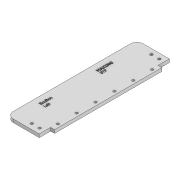
# Autodesk Inventor part: Comb2
Saved by Autodesk Inventor 2020 (Build 240168000, 168)
## iProperties
Created: 2022-04-26
Part Number: Comb2
Material: Generic
Document SubType Name: Modeling
Designer: ferrerx
Density: 1 g/cm^3
Appearance: Default
Author: ferrerx
Autodesk Inventor part; units mm, degrees
ref_plane "YZ Plane" through (0, 0, 0) normal (1, 0, 0) x (0, 1, 0)
ref_plane "XZ Plane" through (0, 0, 0) normal (0, 1, 0) x (-1, 0, 0)
ref_plane "XY Plane" through (0, 0, 0) normal (0, 0, 1) x (1, 0, 0)
sketch "Sketch1" plane through (0, 0, 0) normal (0, 1, 0) x (-1, 0, 0)
  line L0 (25, 100) -> (-25, 100)
  line L1 (-25, 100) -> (-25, -100)
  line L2 (-25, -100) -> (25, -100)
  line L3 (25, -100) -> (25, 100)
  line L4 (25, 100) -> (-25, -100) construction
  line L5 (-25, 100) -> (25, -100) construction
  point P0 (0, 0)
  dimension "d0" = 200
  dimension "d1" = 50
  constraints: 12 end point, 2 midpoint, 2 parallel, 1 horizontal, 1 perpendicular
  measures "d0" distance of L2.end L0.start
  measures "d1" distance of L1.end L2.end
extrude "Extrusion1" add sketch "Sketch1" along normal blind 5
sketch "Sketch2" plane through (0, 5, 0) normal (0, 1, 0) x (1, 0, 0)
  line L0 (0, 0) -> (25, 0) construction
  line L1 (25, -100) -> (25, 100) projected
  line L2 (25, -92) -> (-15.0756, -92) construction
  circle A0 centre (17.5, -92) radius 2
  circle A1 centre (5.5, -92) radius 2
  line L3 (-25, -100) -> (25, -100) projected
  circle A2 centre (17.5, 92) radius 2
  circle A3 centre (5.5, 92) radius 2
  dimension "d4" = 4
  dimension "d5" = 4
  dimension "d6" = 12
  dimension "d7" = 8
  dimension "d10" = 7.5
  constraints: 4 centre point, 4 end point, 3 point on line, 2 symmetric about line, 1 horizontal, 1 midpoint, 2 other
  measures "d4" diameter of A1
  measures "d5" diameter of A0
  measures "d6" distance of A1.centre A0.centre
  measures "d7" distance between parallel lines of L3 L2
  measures "d10" distance from line of L1 A0.centre
extrude "Extrusion2" cut sketch "Sketch2" against normal blind 5
sketch "Sketch3" plane through (0, 5, 0) normal (0, 1, 0) x (1, 0, 0)
  line L0 (19, -82.5) -> (31, -82.5)
  line L1 (31, -82.5) -> (31, 82.5)
  line L2 (31, 82.5) -> (19, 82.5)
  line L3 (19, 82.5) -> (19, -82.5)
  line L4 (25, -100) -> (25, 100) projected
  line L5 (19, -82.5) -> (31, 82.5) construction
  line L6 (31, -82.5) -> (19, 82.5) construction
  point P0 (0, 0)
  point P1 (25, 0)
  dimension "d11" = 165
  dimension "d12" = 12
  constraints: 12 end point, 3 midpoint, 2 parallel, 1 horizontal, 1 perpendicular
  measures "d11" distance of L0.end L1.end
  measures "d12" distance of L1.end L2.end
extrude "Extrusion3" add sketch "Sketch3" against normal blind 5
sketch "Sketch4" plane through (0, 5, 0) normal (0, 1, 0) x (1, 0, 0)
  line L0 (25, -100) -> (25, -82.5) projected
  line L1 (31, 82.5) -> (25, 82.5) projected
  circle A0 centre (26, -72.5) radius 2
  line L2 (25, -82.5) -> (31, -82.5) projected
  line L3 (31, -82.5) -> (31, 82.5) projected
  point P0 (0, 0)
  dimension "d15" = 4
  dimension "d16" = 10
  dimension "d17" = 5
  constraints: 1 centre point
  measures "d15" diameter of A0
  measures "d16" distance from line of L2 A0.centre
  measures "d17" distance from line of L3 A0.centre
extrude "Extrusion4" cut sketch "Sketch4" against normal blind 5
pattern_linear "Rectangular Pattern1" count 6 spacing 29 along (0, 0, -1) of "Extrusion4"
fillet "Fillet1" radius 10 2 edges at (-25, 2.5, -100) (-25, 2.5, 100)
sketch "Sketch5" plane through (0, 5, 0) normal (0, 1, 0) x (1, 0, 0)
  line L0 (14.5574, 78.2537) -> (14.5574, 41.6)
  line L1 (14.5574, 41.6) -> (-22.0963, 41.6)
  line L2 (-22.0963, 41.6) -> (-22.0963, 78.2537)
  line L3 (-22.0963, 60) -> (14.5574, 60)
  line L4 (-22.0387, 23.3375) -> (14.5574, 23.3375)
  line L5 (14.5574, 23.3375) -> (14.5574, 60)
  line L6 (14.5574, 60) -> (-22.0387, 60)
  line L7 (-22.0387, 60) -> (-22.0387, 23.3375)
  line L8 (25, 100) -> (-15, 100) projected
  line L9 (-22.0387, 60) -> (31, 60) construction
  line L10 (31, -82.5) -> (31, 82.5) projected
  line L11 (-12.3449, 32.3329) -> (-12.3449, 31.3043)
  line L12 (-12.3449, 31.3043) -> (-15.0767, 31.3043)
  line L13 (-15.0767, 31.3043) -> (-13.3134, 30.5562)
  line L14 (-13.3134, 30.5562) -> (-13.3134, 29.8482)
  line L15 (-13.3134, 29.8482) -> (-15.0767, 29.1001)
  line L16 (-15.0767, 29.1001) -> (-12.3449, 29.1001)
  line L17 (-12.3449, 29.1001) -> (-12.3449, 28.1249)
  line L18 (-12.3449, 28.1249) -> (-16.466, 28.1249)
  line L19 (-16.466, 28.1249) -> (-16.466, 29.3172)
  line L20 (-16.466, 29.3172) -> (-14.4321, 30.2322)
  line L21 (-14.4321, 30.2322) -> (-16.466, 31.1406)
  line L22 (-16.466, 31.1406) -> (-16.466, 32.3329)
  line L23 (-16.466, 32.3329) -> (-12.3449, 32.3329)
  line L24 (-12.3449, 32.7437) -> (-16.466, 34.1363)
  line L25 (-16.466, 34.1363) -> (-16.466, 35.2651)
  line L26 (-16.466, 35.2651) -> (-12.3449, 36.6578)
  line L27 (-12.3449, 36.6578) -> (-12.3449, 35.5924)
  line L28 (-12.3449, 35.5924) -> (-13.1865, 35.3353)
  line L29 (-13.1865, 35.3353) -> (-13.1865, 34.0395)
  line L30 (-13.1865, 34.0395) -> (-12.3449, 33.779)
  line L31 (-12.3449, 33.779) -> (-12.3449, 32.7437)
  line L32 (-13.9345, 35.1082) -> (-15.2971, 34.6874)
  line L33 (-15.2971, 34.6874) -> (-13.9345, 34.2632)
  line L34 (-13.9345, 34.2632) -> (-13.9345, 35.1082)
  line L35 (-12.3449, 40.6787) -> (-12.3449, 39.4263)
  line L36 (-12.3449, 39.4263) -> (-14.018, 38.3076)
  line L37 (-14.018, 38.3076) -> (-13.7375, 38.1038)
  line L38 (-13.7375, 38.1038) -> (-12.3449, 38.1038)
  line L39 (-12.3449, 38.1038) -> (-12.3449, 37.0685)
  line L40 (-12.3449, 37.0685) -> (-16.466, 37.0685)
  line L41 (-16.466, 37.0685) -> (-16.466, 38.1038)
  line L42 (-16.466, 38.1038) -> (-14.6258, 38.1038)
  line L43 (-14.6258, 38.1038) -> (-16.466, 39.4263)
  line L44 (-16.466, 39.4263) -> (-16.466, 40.6186)
  line L45 (-16.466, 40.6186) -> (-14.5524, 39.1492)
  line L46 (-14.5524, 39.1492) -> (-12.3449, 40.6787)
  line L47 (-12.3449, 43.0666) -> (-12.3449, 40.849)
  line L48 (-12.3449, 40.849) -> (-13.0629, 40.849)
  line L49 (-13.0629, 40.849) -> (-13.0629, 41.4402)
  line L50 (-13.0629, 41.4402) -> (-15.748, 41.4402)
  line L51 (-15.748, 41.4402) -> (-15.748, 40.849)
  line L52 (-15.748, 40.849) -> (-16.466, 40.849)
  line L53 (-16.466, 40.849) -> (-16.466, 43.0666)
  line L54 (-16.466, 43.0666) -> (-15.748, 43.0666)
  line L55 (-15.748, 43.0666) -> (-15.748, 42.4755)
  line L56 (-15.748, 42.4755) -> (-13.0629, 42.4755)
  line L57 (-13.0629, 42.4755) -> (-13.0629, 43.0666)
  line L58 (-13.0629, 43.0666) -> (-12.3449, 43.0666)
  line L59 (-12.3449, 47.2846) -> (-12.3449, 46.2894)
  line L60 (-12.3449, 46.2894) -> (-15.217, 44.6997)
  line L61 (-15.217, 44.6997) -> (-12.3449, 44.6997)
  line L62 (-12.3449, 44.6997) -> (-12.3449, 43.7546)
  line L63 (-12.3449, 43.7546) -> (-16.466, 43.7546)
  line L64 (-16.466, 43.7546) -> (-16.466, 45.0236)
  line L65 (-16.466, 45.0236) -> (-14.1049, 46.3395)
  line L66 (-14.1049, 46.3395) -> (-16.466, 46.3395)
  line L67 (-16.466, 46.3395) -> (-16.466, 47.2846)
  line L68 (-16.466, 47.2846) -> (-12.3449, 47.2846)
  spline S0 degree 2 poles (-12.5786, 51.5627) (-12.4684, 51.2922) (-12.258, 50.4272) (-12.258, 50.0064) knots 0 0 0 1 2 2 2
  spline S1 degree 2 poles (-12.258, 50.0064) (-12.258, 49.0346) (-13.3802, 47.8824) (-14.4088, 47.8824) knots 0 0 0 1 2 2 2
  spline S2 degree 2 poles (-14.4088, 47.8824) (-15.3773, 47.8824) (-16.5462, 49.0346) (-16.5462, 50.0365) knots 0 0 0 1 2 2 2
  spline S3 degree 2 poles (-16.5462, 50.0365) (-16.5462, 50.5541) (-16.3491, 51.202) (-16.1821, 51.546) knots 0 0 0 1 2 2 2
  line L69 (-16.1821, 51.546) -> (-15.2136, 51.546)
  line L70 (-15.2136, 51.546) -> (-15.2136, 51.4525)
  spline S4 degree 2 poles (-15.2136, 51.4525) (-15.2704, 51.379) (-15.4875, 51.0985) (-15.561, 50.9649) knots 0 0 0 1 2 2 2
  spline S5 degree 2 poles (-15.561, 50.9649) (-15.6511, 50.8113) (-15.778, 50.4038) (-15.778, 50.1767) knots 0 0 0 1 2 2 2
  spline S6 degree 2 poles (-15.778, 50.1767) (-15.778, 49.9129) (-15.6111, 49.4754) (-15.4407, 49.3051) knots 0 0 0 1 2 2 2
  spline S7 degree 2 poles (-15.4407, 49.3051) (-15.2737, 49.1414) (-14.7628, 48.9511) (-14.4255, 48.9511) knots 0 0 0 1 2 2 2
  spline S8 degree 2 poles (-14.4255, 48.9511) (-13.7041, 48.9511) (-13.0161, 49.6758) (-13.0161, 50.3003) knots 0 0 0 1 2 2 2
  spline S9 degree 2 poles (-13.0161, 50.3003) (-13.0161, 50.3571) (-13.0228, 50.504) (-13.0261, 50.5608) knots 0 0 0 1 2 2 2
  line L71 (-13.0261, 50.5608) -> (-13.8377, 50.5608)
  line L72 (-13.8377, 50.5608) -> (-13.8377, 49.7626)
  line L73 (-13.8377, 49.7626) -> (-14.6092, 49.7626)
  line L74 (-14.6092, 49.7626) -> (-14.6092, 51.5627)
  line L75 (-14.6092, 51.5627) -> (-12.5786, 51.5627)
  spline S10 degree 2 poles (-6.6136, 29.2163) (-6.6136, 28.7823) (-6.7949, 28.1735) (-6.9245, 27.9047) knots 0 0 0 1 2 2 2
  line L76 (-6.9245, 27.9047) -> (-7.5916, 27.9047)
  line L77 (-7.5916, 27.9047) -> (-7.5916, 27.9436)
  spline S11 degree 2 poles (-7.5916, 27.9436) (-7.3455, 28.2059) (-7.0734, 28.8698) (-7.0734, 29.1774) knots 0 0 0 1 2 2 2
  spline S12 degree 2 poles (-7.0734, 29.1774) (-7.0734, 29.6178) (-7.4394, 30.068) (-7.7406, 30.068) knots 0 0 0 1 2 2 2
  spline S13 degree 2 poles (-7.7406, 30.068) (-7.9802, 30.068) (-8.2782, 29.8316) (-8.3526, 29.5757) knots 0 0 0 1 2 2 2
  spline S14 degree 2 poles (-8.3526, 29.5757) (-8.4045, 29.3912) (-8.4757, 29.0835) (-8.534, 28.8536) knots 0 0 0 1 2 2 2
  spline S15 degree 2 poles (-8.534, 28.8536) (-8.589, 28.6463) (-8.7542, 28.3192) (-8.887, 28.1929) knots 0 0 0 1 2 2 2
  spline S16 degree 2 poles (-8.887, 28.1929) (-9.0198, 28.0699) (-9.376, 27.9338) (-9.6092, 27.9338) knots 0 0 0 1 2 2 2
  spline S17 degree 2 poles (-9.6092, 27.9338) (-10.0949, 27.9338) (-10.7523, 28.6916) (-10.7523, 29.2778) knots 0 0 0 1 2 2 2
  spline S18 degree 2 poles (-10.7523, 29.2778) (-10.7523, 29.6146) (-10.6196, 30.2105) (-10.4933, 30.4663) knots 0 0 0 1 2 2 2
  line L78 (-10.4933, 30.4663) -> (-9.8585, 30.4663)
  line L79 (-9.8585, 30.4663) -> (-9.8585, 30.4275)
  spline S19 degree 2 poles (-9.8585, 30.4275) (-10.0334, 30.2364) (-10.2925, 29.6405) (-10.2925, 29.3134) knots 0 0 0 1 2 2 2
  spline S20 degree 2 poles (-10.2925, 29.3134) (-10.2925, 28.9442) (-9.946, 28.4876) (-9.6642, 28.4876) knots 0 0 0 1 2 2 2
  spline S21 degree 2 poles (-9.6642, 28.4876) (-9.4116, 28.4876) (-9.1104, 28.7564) (-9.0424, 29.009) knots 0 0 0 1 2 2 2
  spline S22 degree 2 poles (-9.0424, 29.009) (-8.9971, 29.1774) (-8.8805, 29.6664) (-8.8319, 29.8283) knots 0 0 0 1 2 2 2
  spline S23 degree 2 poles (-8.8319, 29.8283) (-8.7056, 30.2396) (-8.1972, 30.6218) (-7.8248, 30.6218) knots 0 0 0 1 2 2 2
  spline S24 degree 2 poles (-7.8248, 30.6218) (-7.5884, 30.6218) (-7.135, 30.4307) (-6.9763, 30.2591) knots 0 0 0 1 2 2 2
  spline S25 degree 2 poles (-6.9763, 30.2591) (-6.8014, 30.068) (-6.6136, 29.5822) (-6.6136, 29.2163) knots 0 0 0 1 2 2 2
  line L80 (-6.6848, 32.0953) -> (-10.2083, 32.0953)
  line L81 (-10.2083, 32.0953) -> (-10.2083, 30.7545)
  line L82 (-10.2083, 30.7545) -> (-10.6811, 30.7545)
  line L83 (-10.6811, 30.7545) -> (-10.6811, 33.9671)
  line L84 (-10.6811, 33.9671) -> (-10.2083, 33.9671)
  line L85 (-10.2083, 33.9671) -> (-10.2083, 32.6264)
  line L86 (-10.2083, 32.6264) -> (-6.6848, 32.6264)
  line L87 (-6.6848, 32.6264) -> (-6.6848, 32.0953)
  spline S26 degree 2 poles (-9.4764, 36.8979) (-9.2173, 36.8979) (-8.751, 36.7133) (-8.589, 36.5482) knots 0 0 0 1 2 2 2
  spline S27 degree 2 poles (-8.589, 36.5482) (-8.385, 36.3409) (-8.1745, 35.7806) (-8.1745, 35.3532) knots 0 0 0 1 2 2 2
  line L88 (-8.1745, 35.3532) -> (-8.1745, 34.903)
  line L89 (-8.1745, 34.903) -> (-6.6848, 34.903)
  line L90 (-6.6848, 34.903) -> (-6.6848, 34.3719)
  line L91 (-6.6848, 34.3719) -> (-10.6811, 34.3719)
  line L92 (-10.6811, 34.3719) -> (-10.6811, 35.3758)
  spline S28 degree 2 poles (-10.6811, 35.3758) (-10.6811, 35.7321) (-10.5645, 36.2308) (-10.4317, 36.4219) knots 0 0 0 1 2 2 2
  spline S29 degree 2 poles (-10.4317, 36.4219) (-10.2795, 36.6453) (-9.8099, 36.8979) (-9.4764, 36.8979) knots 0 0 0 1 2 2 2
  spline S30 degree 2 poles (-9.4602, 36.3441) (-9.6675, 36.3441) (-9.9719, 36.2016) (-10.069, 36.0559) knots 0 0 0 1 2 2 2
  spline S31 degree 2 poles (-10.069, 36.0559) (-10.1532, 35.9296) (-10.2212, 35.5928) (-10.2212, 35.3435) knots 0 0 0 1 2 2 2
  line L93 (-10.2212, 35.3435) -> (-10.2212, 34.903)
  line L94 (-10.2212, 34.903) -> (-8.6279, 34.903)
  line L95 (-8.6279, 34.903) -> (-8.6279, 35.2657)
  spline S32 degree 2 poles (-8.6279, 35.2657) (-8.6279, 35.5896) (-8.7315, 35.9879) (-8.8676, 36.1174) knots 0 0 0 1 2 2 2
  spline S33 degree 2 poles (-8.8676, 36.1174) (-8.9874, 36.2373) (-9.2691, 36.3441) (-9.4602, 36.3441) knots 0 0 0 1 2 2 2
  point P0 (0, 0)
  point P1 (-12.258, 27.6974)
  point P2 (-6.6136, 27.6974)
  dimension "d33" = 40
  constraints: 18 end point, 2 horizontal, 2 parallel, 1 perpendicular, 1 point on line, 2 other
  measures "d33" distance between parallel lines of L8 L3
emboss "Emboss1" sketch "Sketch5" operation cut depth 1 direction (0, -1, 0) contours L47 L48 L49 L50 L51 L52 L53 L1 | L1 L53 L54 L55 L56 L57 L58 L47 | L11 L12 L13 L14 L15 L16 L17 L18 L19 L20 L21 L22 L23 | L24 L25 L26 L27 L28 L29 L30 L31 | L35 L36 L37 L38 L39 L40 L41 L42 L43 L44 L45 L46 | L59 L60 L61 L62 L63 L64 L65 L66 L67 L68 | S0 S1 S2 S3 L69 L70 S4 S5 S6 S7 S8 S9 L71 L72 L73 L74 L75 | S10 L76 L77 S11 S12 S13 S14 S15 S16 S17 S18 L78 L79 S19 S20 S21 S22 S23 S24 S25 | L80 L81 L82 L83 L84 L85 L86 L87 | S26 S27 L88 L89 L90 L91 L92 S28 S29
sketch "Sketch6" plane through (0, 5, 0) normal (0, 1, 0) x (1, 0, 0)
  line L0 (-16.466, -60) -> (-16.394, -19.5573) construction
  line L1 (-16.394, -19.5573) -> (0.0633, -19.5866) construction
  line L2 (0.0633, -19.5866) -> (-0.0087, -60.0293) construction
  line L3 (-0.0087, -60.0293) -> (-16.466, -60) construction
  line L4 (-12.3449, 28.1249) -> (-16.466, 28.1249) projected
  line L5 (-16.466, -60) -> (-16.466, 28.1249) construction
  line L6 (31, -82.5) -> (31, 82.5) projected
  line L7 (-15, -100) -> (25, -100) projected
  line L8 (-16.466, -60) -> (31, -60) construction
  spline S0 degree 2 poles (-13.5135, -56.8898) (-13.2155, -56.8904) (-12.7593, -57.1179) (-12.6107, -57.306) knots 0 0 0 1 2 2 2
  spline S1 degree 2 poles (-12.6107, -57.306) (-12.4362, -57.533) (-12.2881, -58.0482) (-12.2889, -58.4562) knots 0 0 0 1 2 2 2
  line L9 (-12.2889, -58.4562) -> (-12.2909, -59.6026)
  line L10 (-12.2909, -59.6026) -> (-16.2872, -59.5955)
  line L11 (-16.2872, -59.5955) -> (-16.2853, -58.5365)
  spline S2 degree 2 poles (-16.2853, -58.5365) (-16.2845, -58.1091) (-16.2287, -57.6817) (-16.1215, -57.4876) knots 0 0 0 1 2 2 2
  spline S3 degree 2 poles (-16.1215, -57.4876) (-16.0078, -57.2708) (-15.635, -57.0739) (-15.3824, -57.0744) knots 0 0 0 1 2 2 2
  spline S4 degree 2 poles (-15.3824, -57.0744) (-15.1006, -57.0749) (-14.6543, -57.3736) (-14.5284, -57.6361) knots 0 0 0 1 2 2 2
  line L12 (-14.5284, -57.6361) -> (-14.509, -57.6362)
  spline S5 degree 2 poles (-14.509, -57.6362) (-14.4112, -57.2801) (-13.8956, -56.8892) (-13.5135, -56.8898) knots 0 0 0 1 2 2 2
  spline S6 degree 2 poles (-13.4918, -57.4437) (-13.7185, -57.4433) (-14.0102, -57.5723) (-14.1141, -57.7664) knots 0 0 0 1 2 2 2
  spline S7 degree 2 poles (-14.1141, -57.7664) (-14.1791, -57.8926) (-14.2185, -58.1905) (-14.219, -58.4657) knots 0 0 0 1 2 2 2
  line L13 (-14.219, -58.4657) -> (-14.2201, -59.0681)
  line L14 (-14.2201, -59.0681) -> (-12.7433, -59.0707)
  line L15 (-12.7433, -59.0707) -> (-12.7426, -58.64)
  spline S8 degree 2 poles (-12.7426, -58.64) (-12.742, -58.2902) (-12.806, -57.8886) (-12.9094, -57.7329) knots 0 0 0 1 2 2 2
  spline S9 degree 2 poles (-12.9094, -57.7329) (-13.016, -57.5838) (-13.2813, -57.444) (-13.4918, -57.4437) knots 0 0 0 1 2 2 2
  spline S10 degree 2 poles (-15.3089, -57.6283) (-15.4514, -57.628) (-15.6653, -57.7248) (-15.727, -57.8315) knots 0 0 0 1 2 2 2
  spline S11 degree 2 poles (-15.727, -57.8315) (-15.7985, -57.961) (-15.8314, -58.275) (-15.8319, -58.5568) knots 0 0 0 1 2 2 2
  line L16 (-15.8319, -58.5568) -> (-15.8328, -59.0652)
  line L17 (-15.8328, -59.0652) -> (-14.6638, -59.0673)
  line L18 (-14.6638, -59.0673) -> (-14.6627, -58.4649)
  spline S12 degree 2 poles (-14.6627, -58.4649) (-14.6622, -58.2156) (-14.7136, -57.9791) (-14.7944, -57.8526) knots 0 0 0 1 2 2 2
  spline S13 degree 2 poles (-14.7944, -57.8526) (-14.8719, -57.7294) (-15.1211, -57.6286) (-15.3089, -57.6283) knots 0 0 0 1 2 2 2
  spline S14 degree 2 poles (-13.7802, -53.9359) (-13.0224, -53.9372) (-12.1979, -54.6674) (-12.199, -55.2762) knots 0 0 0 1 2 2 2
  spline S15 degree 2 poles (-12.199, -55.2762) (-12.2001, -55.9012) (-13.0531, -56.6154) (-13.785, -56.6141) knots 0 0 0 1 2 2 2
  spline S16 degree 2 poles (-13.785, -56.6141) (-14.5363, -56.6128) (-15.3673, -55.8729) (-15.3662, -55.2706) knots 0 0 0 1 2 2 2
  spline S17 degree 2 poles (-15.3662, -55.2706) (-15.3651, -54.6617) (-14.5348, -53.9345) (-13.7802, -53.9359) knots 0 0 0 1 2 2 2
  spline S18 degree 2 poles (-13.7812, -54.4573) (-14.3641, -54.4562) (-14.9316, -54.8795) (-14.9323, -55.2713) knots 0 0 0 1 2 2 2
  spline S19 degree 2 poles (-14.9323, -55.2713) (-14.933, -55.6632) (-14.367, -56.0917) (-13.7841, -56.0927) knots 0 0 0 1 2 2 2
  spline S20 degree 2 poles (-13.7841, -56.0927) (-13.2173, -56.0937) (-12.6337, -55.6673) (-12.633, -55.2754) knots 0 0 0 1 2 2 2
  spline S21 degree 2 poles (-12.633, -55.2754) (-12.6323, -54.8868) (-13.2047, -54.4583) (-13.7812, -54.4573) knots 0 0 0 1 2 2 2
  line L19 (-12.2758, -51.0887) -> (-12.2767, -51.5939)
  line L20 (-12.2767, -51.5939) -> (-12.607, -51.5933)
  spline S22 degree 2 poles (-12.607, -51.5933) (-12.4034, -51.8269) (-12.1936, -52.245) (-12.1941, -52.5041) knots 0 0 0 1 2 2 2
  spline S23 degree 2 poles (-12.1941, -52.5041) (-12.1944, -52.6984) (-12.3246, -53.0447) (-12.4641, -53.1707) knots 0 0 0 1 2 2 2
  spline S24 degree 2 poles (-12.4641, -53.1707) (-12.6035, -53.3) (-13.028, -53.4417) (-13.3324, -53.4412) knots 0 0 0 1 2 2 2
  line L21 (-13.3324, -53.4412) -> (-15.2788, -53.4377)
  line L22 (-15.2788, -53.4377) -> (-15.2779, -52.9325)
  line L23 (-15.2779, -52.9325) -> (-13.568, -52.9356)
  spline S25 degree 2 poles (-13.568, -52.9356) (-13.3283, -52.936) (-13.0141, -52.9009) (-12.8974, -52.8396) knots 0 0 0 1 2 2 2
  spline S26 degree 2 poles (-12.8974, -52.8396) (-12.7807, -52.7783) (-12.6735, -52.568) (-12.6731, -52.3704) knots 0 0 0 1 2 2 2
  spline S27 degree 2 poles (-12.6731, -52.3704) (-12.6728, -52.1858) (-12.8826, -51.7677) (-13.0345, -51.5926) knots 0 0 0 1 2 2 2
  line L24 (-13.0345, -51.5926) -> (-15.2755, -51.5886)
  line L25 (-15.2755, -51.5886) -> (-15.2746, -51.0834)
  line L26 (-15.2746, -51.0834) -> (-12.2758, -51.0887)
  line L27 (-12.2735, -49.8419) -> (-12.2744, -50.3471)
  line L28 (-12.2744, -50.3471) -> (-16.4488, -50.3397)
  line L29 (-16.4488, -50.3397) -> (-16.4479, -49.8345)
  line L30 (-16.4479, -49.8345) -> (-12.2735, -49.8419)
  spline S28 degree 2 poles (-12.2123, -48.1936) (-12.213, -48.6049) (-12.6834, -49.0672) (-13.1919, -49.0663) knots 0 0 0 1 2 2 2
  line L31 (-13.1919, -49.0663) -> (-14.8532, -49.0633)
  line L32 (-14.8532, -49.0633) -> (-14.8538, -49.4034)
  line L33 (-14.8538, -49.4034) -> (-15.2716, -49.4026)
  line L34 (-15.2716, -49.4026) -> (-15.271, -49.0626)
  line L35 (-15.271, -49.0626) -> (-16.1324, -49.061)
  line L36 (-16.1324, -49.061) -> (-16.1315, -48.5558)
  line L37 (-16.1315, -48.5558) -> (-15.2701, -48.5574)
  line L38 (-15.2701, -48.5574) -> (-15.2684, -47.6279)
  line L39 (-15.2684, -47.6279) -> (-14.8507, -47.6287)
  line L40 (-14.8507, -47.6287) -> (-14.8523, -48.5581)
  line L41 (-14.8523, -48.5581) -> (-13.4242, -48.5607)
  spline S29 degree 2 poles (-13.4242, -48.5607) (-13.1975, -48.5611) (-12.9481, -48.5453) (-12.8411, -48.4904) knots 0 0 0 1 2 2 2
  spline S30 degree 2 poles (-12.8411, -48.4904) (-12.7471, -48.4453) (-12.6528, -48.2414) (-12.6525, -48.0665) knots 0 0 0 1 2 2 2
  spline S31 degree 2 poles (-12.6525, -48.0665) (-12.6523, -47.9435) (-12.7264, -47.7134) (-12.749, -47.6616) knots 0 0 0 1 2 2 2
  line L42 (-12.749, -47.6616) -> (-12.7489, -47.6324)
  line L43 (-12.7489, -47.6324) -> (-12.2955, -47.6332)
  spline S32 degree 2 poles (-12.2955, -47.6332) (-12.2569, -47.7758) (-12.2121, -48.0673) (-12.2123, -48.1936) knots 0 0 0 1 2 2 2
  spline S33 degree 2 poles (-13.764, -44.7937) (-13.0062, -44.7951) (-12.1817, -45.5252) (-12.1827, -46.134) knots 0 0 0 1 2 2 2
  spline S34 degree 2 poles (-12.1827, -46.134) (-12.1839, -46.759) (-13.0368, -47.4732) (-13.7687, -47.4719) knots 0 0 0 1 2 2 2
  spline S35 degree 2 poles (-13.7687, -47.4719) (-14.5201, -47.4706) (-15.351, -46.7307) (-15.35, -46.1284) knots 0 0 0 1 2 2 2
  spline S36 degree 2 poles (-15.35, -46.1284) (-15.3489, -45.5195) (-14.5185, -44.7924) (-13.764, -44.7937) knots 0 0 0 1 2 2 2
  spline S37 degree 2 poles (-13.7649, -45.3151) (-14.3478, -45.3141) (-14.9153, -45.7373) (-14.916, -46.1291) knots 0 0 0 1 2 2 2
  spline S38 degree 2 poles (-14.916, -46.1291) (-14.9167, -46.521) (-14.3507, -46.9495) (-13.7678, -46.9505) knots 0 0 0 1 2 2 2
  spline S39 degree 2 poles (-13.7678, -46.9505) (-13.2011, -46.9515) (-12.6174, -46.5251) (-12.6167, -46.1332) knots 0 0 0 1 2 2 2
  spline S40 degree 2 poles (-12.6167, -46.1332) (-12.616, -45.7446) (-13.1885, -45.3161) (-13.7649, -45.3151) knots 0 0 0 1 2 2 2
  line L44 (-12.2595, -41.9239) -> (-12.2603, -42.4291)
  line L45 (-12.2603, -42.4291) -> (-13.9703, -42.426)
  spline S41 degree 2 poles (-13.9703, -42.426) (-14.1775, -42.4257) (-14.5338, -42.4639) (-14.6408, -42.522) knots 0 0 0 1 2 2 2
  spline S42 degree 2 poles (-14.6408, -42.522) (-14.7542, -42.5833) (-14.8647, -42.8033) (-14.8651, -42.9912) knots 0 0 0 1 2 2 2
  spline S43 degree 2 poles (-14.8651, -42.9912) (-14.8654, -43.179) (-14.6653, -43.5777) (-14.5038, -43.769) knots 0 0 0 1 2 2 2
  line L46 (-14.5038, -43.769) -> (-12.2627, -43.773)
  line L47 (-12.2627, -43.773) -> (-12.2636, -44.2782)
  line L48 (-12.2636, -44.2782) -> (-15.2625, -44.2729)
  line L49 (-15.2625, -44.2729) -> (-15.2616, -43.7677)
  line L50 (-15.2616, -43.7677) -> (-14.928, -43.7683)
  spline S44 degree 2 poles (-14.928, -43.7683) (-15.1316, -43.5412) (-15.3446, -43.1037) (-15.3441, -42.8575) knots 0 0 0 1 2 2 2
  spline S45 degree 2 poles (-15.3441, -42.8575) (-15.3434, -42.4171) (-14.7595, -41.9194) (-14.2058, -41.9204) knots 0 0 0 1 2 2 2
  line L51 (-14.2058, -41.9204) -> (-12.2595, -41.9239)
  line L52 (-5.7071, -57.2988) -> (-5.7112, -59.6143)
  line L53 (-5.7112, -59.6143) -> (-9.7074, -59.6072)
  line L54 (-9.7074, -59.6072) -> (-9.7065, -59.0761)
  line L55 (-9.7065, -59.0761) -> (-6.183, -59.0824)
  line L56 (-6.183, -59.0824) -> (-6.1799, -57.298)
  line L57 (-6.1799, -57.298) -> (-5.7071, -57.2988)
  spline S46 degree 2 poles (-6.0208, -55.2483) (-5.9755, -55.3099) (-5.814, -55.5175) (-5.7656, -55.6147) knots 0 0 0 1 2 2 2
  spline S47 degree 2 poles (-5.7656, -55.6147) (-5.6946, -55.7476) (-5.6205, -55.9971) (-5.6209, -56.2238) knots 0 0 0 1 2 2 2
  spline S48 degree 2 poles (-5.6209, -56.2238) (-5.6213, -56.4084) (-5.7611, -56.7417) (-5.8876, -56.8678) knots 0 0 0 1 2 2 2
  spline S49 degree 2 poles (-5.8876, -56.8678) (-6.0109, -56.9874) (-6.3739, -57.1325) (-6.5747, -57.1321) knots 0 0 0 1 2 2 2
  spline S50 degree 2 poles (-6.5747, -57.1321) (-6.8856, -57.1316) (-7.3255, -56.8685) (-7.4513, -56.5833) knots 0 0 0 1 2 2 2
  spline S51 degree 2 poles (-7.4513, -56.5833) (-7.5674, -56.3305) (-7.6537, -55.6437) (-7.6756, -55.2454) knots 0 0 0 1 2 2 2
  line L58 (-7.6756, -55.2454) -> (-7.7728, -55.2452)
  spline S52 degree 2 poles (-7.7728, -55.2452) (-7.9477, -55.2449) (-8.1648, -55.3514) (-8.2265, -55.4484) knots 0 0 0 1 2 2 2
  spline S53 degree 2 poles (-8.2265, -55.4484) (-8.2882, -55.5455) (-8.3276, -55.8239) (-8.3279, -55.9729) knots 0 0 0 1 2 2 2
  spline S54 degree 2 poles (-8.3279, -55.9729) (-8.3282, -56.1477) (-8.2254, -56.6207) (-8.1254, -56.8573) knots 0 0 0 1 2 2 2
  line L59 (-8.1254, -56.8573) -> (-8.1255, -56.8865)
  line L60 (-8.1255, -56.8865) -> (-8.6404, -56.8856)
  spline S55 degree 2 poles (-8.6404, -56.8856) (-8.679, -56.7462) (-8.7752, -56.2247) (-8.7748, -55.9688) knots 0 0 0 1 2 2 2
  spline S56 degree 2 poles (-8.7748, -55.9688) (-8.7742, -55.6579) (-8.6763, -55.2339) (-8.5497, -55.0657) knots 0 0 0 1 2 2 2
  spline S57 degree 2 poles (-8.5497, -55.0657) (-8.4263, -54.9008) (-8.0342, -54.7395) (-7.7525, -54.74) knots 0 0 0 1 2 2 2
  line L61 (-7.7525, -54.74) -> (-5.7025, -54.7437)
  line L62 (-5.7025, -54.7437) -> (-5.7034, -55.2489)
  line L63 (-5.7034, -55.2489) -> (-6.0208, -55.2483)
  line L64 (-6.4418, -55.2476) -> (-7.2741, -55.2461)
  spline S58 degree 2 poles (-7.2741, -55.2461) (-7.2582, -55.4275) (-7.2041, -55.9749) (-7.1526, -56.1466) knots 0 0 0 1 2 2 2
  spline S59 degree 2 poles (-7.1526, -56.1466) (-7.0914, -56.3475) (-6.8361, -56.6103) (-6.6094, -56.6107) knots 0 0 0 1 2 2 2
  spline S60 degree 2 poles (-6.6094, -56.6107) (-6.3503, -56.6111) (-6.0874, -56.3201) (-6.087, -56.0416) knots 0 0 0 1 2 2 2
  spline S61 degree 2 poles (-6.087, -56.0416) (-6.0865, -55.8052) (-6.2899, -55.4162) (-6.4418, -55.2476) knots 0 0 0 1 2 2 2
  spline S62 degree 2 poles (-7.2448, -51.5187) (-6.5096, -51.52) (-5.6138, -52.234) (-5.6148, -52.7716) knots 0 0 0 1 2 2 2
  spline S63 degree 2 poles (-5.6148, -52.7716) (-5.6152, -53.0145) (-5.7357, -53.3608) (-5.8396, -53.529) knots 0 0 0 1 2 2 2
  line L65 (-5.8396, -53.529) -> (-5.7004, -53.5616)
  line L66 (-5.7004, -53.5616) -> (-5.7012, -54.0345)
  line L67 (-5.7012, -54.0345) -> (-9.8756, -54.027)
  line L68 (-9.8756, -54.027) -> (-9.8747, -53.5218)
  line L69 (-9.8747, -53.5218) -> (-8.385, -53.5245)
  spline S64 degree 2 poles (-8.385, -53.5245) (-8.5563, -53.3331) (-8.7822, -52.889) (-8.7817, -52.6073) knots 0 0 0 1 2 2 2
  spline S65 degree 2 poles (-8.7817, -52.6073) (-8.7808, -52.0989) (-7.9669, -51.5174) (-7.2448, -51.5187) knots 0 0 0 1 2 2 2
  spline S66 degree 2 poles (-7.2068, -52.0401) (-7.7444, -52.0392) (-8.302, -52.3653) (-8.3026, -52.728) knots 0 0 0 1 2 2 2
  spline S67 degree 2 poles (-8.3026, -52.728) (-8.303, -52.932) (-8.1095, -53.3533) (-7.9608, -53.5252) knots 0 0 0 1 2 2 2
  line L70 (-7.9608, -53.5252) -> (-6.2412, -53.5283)
  spline S68 degree 2 poles (-6.2412, -53.5283) (-6.1469, -53.3374) (-6.0687, -53.0428) (-6.0684, -52.868) knots 0 0 0 1 2 2 2
  spline S69 degree 2 poles (-6.0684, -52.868) (-6.0677, -52.4826) (-6.6142, -52.0412) (-7.2068, -52.0401) knots 0 0 0 1 2 2 2
  point P0 (0, 0)
  dimension "d32" = 40
  constraints: 4 end point, 1 horizontal, 1 parallel, 1 point on line, 2 other
  measures "d32" distance between parallel lines of L7 L8
emboss "Emboss2" sketch "Sketch6" operation cut depth 1 direction (0, -1, 0)
body "Solid1"
